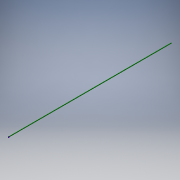
# Autodesk Inventor part: wire
Saved by Autodesk Inventor 2016 SP1 (Build 200210100, 210)
## iProperties
Created: 2017-07-05
Part Number: wire
Material: Типовые
Document SubType Name: Modeling
Designer: user
Density: 1 g/cm^3
Appearance: По умолчанию
Author: user
Autodesk Inventor part; units mm, degrees
ref_plane "YZ Plane" through (0, 0, 0) normal (1, 0, 0) x (0, 1, 0)
ref_plane "XZ Plane" through (0, 0, 0) normal (0, 1, 0) x (-1, 0, 0)
ref_plane "XY Plane" through (0, 0, 0) normal (0, 0, 1) x (1, 0, 0)
sketch "Эскиз1" plane through (0, 0, 0) normal (0, 1, 0) x (-1, 0, 0)
  circle A0 centre (0, 0) radius 4.4
  circle A1 centre (0, 0) radius 3.4
  circle A2 centre (0, 0) radius 3
  dimension "d0" = 8.8
  dimension "d3" = 6.8
  dimension "d8" = 6
  constraints: 3 centre point, 3 coincident
  measures "d0" diameter of A0
  measures "d3" diameter of A1
  measures "d8" diameter of A2
extrude "Выдавливание4" add sketch "Эскиз1" along normal blind 2000 contours A2
extrude "Выдавливание5" add sketch "Эскиз1" along normal blind 2000 contours A0
